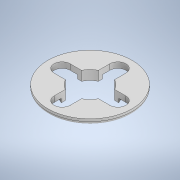
# Autodesk Inventor part: wheel_chain_guide_holes
Saved by Autodesk Inventor 2021 (Build 250183000, 183)
## iProperties
Created: 2021-08-01
Part Number: wheel_chain_guide_holes
Material: Generic
Document SubType Name: Modeling
Designer: Mateusz
Density: 1 g/cm^3
Appearance: Default
Author: Mateusz
Autodesk Inventor part; units mm, degrees
ref_plane "YZ Plane" through (0, 0, 0) normal (1, 0, 0) x (0, 1, 0)
ref_plane "XZ Plane" through (0, 0, 0) normal (0, 1, 0) x (-1, 0, 0)
ref_plane "XY Plane" through (0, 0, 0) normal (0, 0, 1) x (1, 0, 0)
sketch "Sketch1" plane through (0, 0, 0) normal (0, 1, 0) x (-1, 0, 0)
  circle A0 centre (0, 0) radius 52
  circle A1 centre (0, 0) radius 22.75
  circle A2 centre (0, 0) radius 27.5
  dimension "d2" = 45.5
  dimension "d4" = 55
  constraints: 3 centre point, 2 coincident
  measures "d2" diameter of A1
  measures "d4" diameter of A2
extrude "Extrusion1" add sketch "Sketch1" against normal blind 4.75 contours A2
extrude "Extrusion2" add sketch "Sketch1" along normal blind 7 contours A0 | A2
fillet "Fillet1" radius 4 1 edges at (52, 0, 0)
sketch "Sketch2" plane through (0, 7, 0) normal (0, 1, 0) x (1, 0, 0)
  circle A0 centre (34.5, 0) radius 10
  circle A1 centre (0, 34.5) radius 10
  circle A2 centre (-34.5, 0) radius 10
  circle A3 centre (0, -34.5) radius 10
  circle A4 centre (0, 0) radius 52
  line L0 (0, 0) -> (44.5, 0)
  circle A5 centre (0, 0) radius 44.5
  dimension "d14" = 360
  constraints: 4 centre point, 2 coincident, 2 end point, 2 horizontal alignment, 1 horizontal, 13 other
extrude "Extrusion3" cut sketch "Sketch2" against normal through all contours L0 A0 | A0 L0 | A1 | A2 | A3
sketch "Sketch3" plane through (0, 7, 0) normal (0, 1, 0) x (1, 0, 0)
  circle A0 centre (0, 34.5) radius 10 projected
  arc A1 (6.3329, 26.7609) -> (-6.3329, 26.7609) centre (0, 34.5) ccw projected
  line L0 (-10, 34.5) -> (-10, 20.4343)
  circle A2 centre (0, 0) radius 22.75 projected
  line L1 (10, 34.5) -> (10, 20.4343)
  line L2 (-34.5, -10) -> (-20.4343, -10)
  line L3 (-34.5, 10) -> (-20.4343, 10)
  line L4 (10, -34.5) -> (10, -20.4343)
  line L5 (-10, -34.5) -> (-10, -20.4343)
  line L6 (34.5, 10) -> (20.4343, 10)
  line L7 (34.5, -10) -> (20.4343, -10)
  circle A3 centre (-34.5, 0) radius 10 projected
  circle A4 centre (34.5, 0) radius 10 projected
  circle A5 centre (0, -34.5) radius 10 projected
  point P0 (-26.7609, 6.3329)
  point P1 (-26.7609, -6.3329)
  point P2 (-6.3329, -26.7609)
  point P3 (6.3329, -26.7609)
  point P4 (34.5, 0)
  point P5 (26.7609, -6.3329)
  point P6 (26.7609, 6.3329)
  point P7 (34.5, 0)
  dimension "d22" = 360
  constraints: 16 end point, 2 point on circle, 2 vertical, 43 other
extrude "Extrusion5" cut sketch "Sketch3" against normal through all contours L1 A2 L0 A0 | L6 A4 L7 A2 | A2 L2 A3 L3 | A2 L4 A5 L5
body "Solid1"
